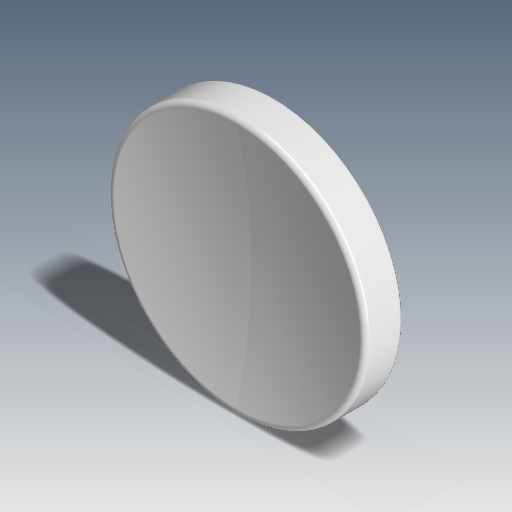
# Autodesk Inventor part: Bi Concave Lens
Saved by Autodesk Inventor 2026 (Build 300175050, 175E)
## iProperties
Created: 2025-08-02
Part Number: Bi Concave Lens
Material: Generic
Document SubType Name: Modeling
Designer: aman0
Density: 1 g/cm^3
Appearance: Default
Author: aman0
Autodesk Inventor part; units mm, degrees
ref_plane "YZ Plane" through (0, 0, 0) normal (1, 0, 0) x (0, 1, 0)
ref_plane "XZ Plane" through (0, 0, 0) normal (0, 1, 0) x (-1, 0, 0)
ref_plane "XY Plane" through (0, 0, 0) normal (0, 0, 1) x (1, 0, 0)
sketch "Sketch1" plane through (0, 0, 0) normal (0, 1, 0) x (-1, 0, 0)
  line L0 (12.5, 2) -> (12.5, -2)
  line L1 (12.5, -2) -> (-12.5, -2)
  line L2 (-12.5, -2) -> (-12.5, 2)
  line L3 (-12.5, 2) -> (12.5, 2)
  circle A0 centre (0, -52) radius 51.5388
  circle A1 centre (0, 52) radius 51.5388
  line L4 (0, 0.4612) -> (0, -0.4612)
  point P0 (0, 0)
  point P1 (12.5, 0)
  point P2 (0, -2)
  point P3 (0, 2)
  dimension "d5" = 25
  dimension "d6" = 4
  dimension "d7" = 50
  dimension "d8" = 50
  constraints: 10 end point, 6 point on circle, 3 midpoint, 2 centre point, 2 parallel, 2 vertical, 1 horizontal alignment, 1 perpendicular, 1 vertical alignment
  measures "d5" distance of L0.end L1.end
  measures "d6" distance of L0.start L0.end
  measures "d7" distance of point (0, -2) A0.centre
  measures "d8" distance of point (0, 2) A1.centre
revolve "Revolution1" add sketch "Sketch1" angle 360 about axis through (0, 0, 0.4612) along (0, 0, -1) contours A1 L4 A0 L2
fillet "Fillet1" radius 0.5 2 edges at (-12.5, 0, 2) (-12.5, 0, -2)
body "Solid1"
